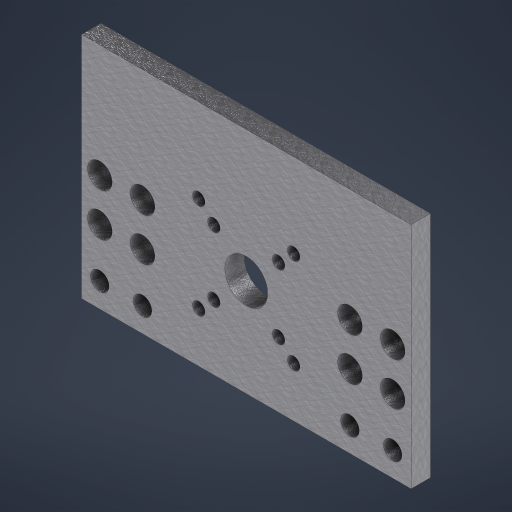
# Autodesk Inventor part: FirstStageMotorPlate
Saved by Autodesk Inventor 2024 (Build 280153000, 153)
## iProperties
Created: 2023-11-22
Part Number: FirstStageMotorPlate
Material: Generic
Document SubType Name: Modeling
Designer: avsar
Density: 1 g/cm^3
Appearance: Machined 02
Author: avsar
Autodesk Inventor part; units mm, degrees
ref_plane "YZ Plane" through (0, 0, 0) normal (1, 0, 0) x (0, 1, 0)
ref_plane "XZ Plane" through (0, 0, 0) normal (0, 1, 0) x (-1, 0, 0)
ref_plane "XY Plane" through (0, 0, 0) normal (0, 0, 1) x (1, 0, 0)
sketch "Sketch1" plane through (0, 0, 0) normal (0, 0, 1) x (1, 0, 0)
  line L0 (-54, -37.5) -> (54, -37.5)
  line L1 (54, -37.5) -> (54, 37.5)
  line L2 (54, 37.5) -> (-54, 37.5)
  line L3 (-54, 37.5) -> (-54, -37.5)
  line L4 (-54, -37.5) -> (54, 37.5) construction
  line L5 (54, -37.5) -> (-54, 37.5) construction
  point P0 (0, 0)
  dimension "d0" = 108
  dimension "d1" = 75
  constraints: 12 end point, 2 midpoint, 2 parallel, 1 horizontal, 1 perpendicular
  measures "d0" distance of L2.end L1.end
  measures "d1" distance of L1.end L0.end
extrude "Extrusion1" add sketch "Sketch1" along normal mid plane 6.35
sketch "Sketch3" plane through (0, 0, 3.175) normal (0, 0, 1) x (1, 0, 0)
  circle A0 centre (0, -5.5) radius 7
  line L0 (-54, -37.5) -> (54, -37.5) projected
  circle A1 centre (-10.6066, 5.1066) radius 2
  line L1 (0, -5.5) -> (-54, -5.5) construction
  line L2 (-54, -37.5) -> (-54, 37.5) construction
  line L3 (0, -5.5) -> (-10.6066, 5.1066) construction
  circle A2 centre (-10.6066, -16.1066) radius 2
  circle A3 centre (10.6066, -16.1066) radius 2
  circle A4 centre (10.6066, 5.1066) radius 2
  line L4 (0, -5.5) -> (-15.5563, 10.0563) construction
  circle A5 centre (-15.5563, 10.0563) radius 2
  circle A6 centre (-15.5563, -21.0563) radius 2
  circle A7 centre (15.5563, -21.0563) radius 2
  circle A8 centre (15.5563, 10.0563) radius 2
  point P0 (0, 0)
  point P1 (0, -37.5)
  dimension "d16" = 14
  dimension "d17" = 32
  dimension "d18" = 4
  dimension "d19" = 45
  dimension "d20" = 15
  dimension "d23" = 360
  dimension "d25" = 22
  dimension "d26" = 4
  dimension "d29" = 360
  constraints: 9 centre point, 6 end point, 1 coincident, 1 collinear, 1 horizontal, 1 midpoint, 1 point on line, 1 vertical alignment, 18 other
  measures "d16" diameter of A0
  measures "d17" distance of point (0, -37.5) L1.start
  measures "d18" diameter of A1
  measures "d19" angle of L1 L3
  measures "d20" distance of L1.start L3.end
  measures "d25" distance of L1.start L4.end
  measures "d26" diameter of A5
extrude "Extrusion3" cut sketch "Sketch3" against normal through all
sketch "Sketch5" plane through (0, 0, 3.175) normal (0, 0, 1) x (1, 0, 0)
  circle A0 centre (-48, -29.5) radius 3
  line L0 (-54, 37.5) -> (-54, -37.5) construction
  line L1 (-54, -37.5) -> (54, -37.5) construction
  circle A1 centre (-34, -29.5) radius 3
  circle A2 centre (-34, -13.5) radius 4
  circle A3 centre (-48, -13.5) radius 4
  circle A4 centre (-34, 0.5) radius 4
  circle A5 centre (-48, 0.5) radius 4
  line L2 (-54, 37.5) -> (54, 37.5) projected
  line L3 (0, 37.5) -> (0, -37.5) construction
  line L4 (54, -37.5) -> (-54, -37.5) construction
  circle A6 centre (48, -29.5) radius 3
  circle A7 centre (34, -29.5) radius 3
  circle A8 centre (34, -13.5) radius 4
  circle A9 centre (48, -13.5) radius 4
  circle A10 centre (34, 0.5) radius 4
  circle A11 centre (48, 0.5) radius 4
  point P0 (0, 0)
  dimension "d45" = 6
  dimension "d46" = 6
  dimension "d47" = 8
  dimension "d48" = 6
  dimension "d49" = 14
  dimension "d50" = 8
  dimension "d51" = 16
  dimension "d52" = 8
  dimension "d53" = 8
  dimension "d54" = 14
  dimension "d55" = 8
  constraints: 12 centre point, 6 symmetric about line, 4 vertical alignment, 3 horizontal alignment, 2 end point, 2 midpoint, 6 other
  measures "d45" diameter of A0
  measures "d46" distance from line of L0 A0.centre
  measures "d47" distance from line of L1 A0.centre
  measures "d48" diameter of A1
  measures "d49" distance of A0.centre A1.centre
  measures "d50" diameter of A2
  measures "d51" distance of A1.centre A2.centre
  measures "d52" diameter of A3
  measures "d53" diameter of A4
  measures "d54" distance of A2.centre A4.centre
  measures "d55" diameter of A5
extrude "Extrusion5" cut sketch "Sketch5" against normal through all
body "Solid1"
